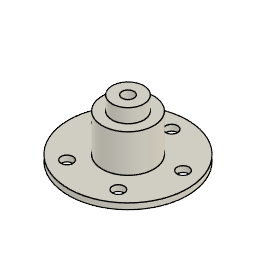
Brodie Stem Bolt (Autodesk Fusion 360 design; units mm, degrees)
Autodesk Fusion 360 part; units mm, degrees
sketch "Sketch1" plane through (0, 0, 0) normal (0, 0, 1) x (1, 0, 0)
  circle A0 centre (0, 0) radius 15
  constraint coincident A0.centre origin
extrude "Extrude1" add sketch "Sketch1" along normal blind 2
sketch "Sketch2" plane through (0, 0, 2) normal (0, 0, 1) x (-1, 0, 0)
  circle A0 centre (0, 0) radius 15
  circle A1 centre (0, -11) radius 1.5
  circle A2 centre (10.4616, -3.3992) radius 1.5
  circle A3 centre (6.4656, 8.8992) radius 1.5
  circle A4 centre (-6.4656, 8.8992) radius 1.5
  circle A5 centre (-10.4616, -3.3992) radius 1.5
  dimension "d4" = 360
extrude "Extrude2" cut sketch "Sketch2" against normal blind 19 contours A1 | A2 | A3 | A4 | A5
sketch "Sketch3" plane through (0, 0, 2) normal (0, 0, 1) x (-1, 0, 0)
  circle A0 centre (6.4656, 8.8992) radius 1.5
  circle A1 centre (10.4616, -3.3992) radius 1.5
  circle A2 centre (-6.4656, 8.8992) radius 1.5
  circle A3 centre (0, -11) radius 1.5
  circle A4 centre (-10.4616, -3.3992) radius 1.5
  circle A5 centre (0, 0) radius 15
  circle A6 centre (0, 0) radius 3
  constraint concentric A5 A6
extrude "Extrude3" cut sketch "Sketch3" against normal blind 2 contours A6
sketch "Sketch4" plane through (0, 0, 2) normal (0, 0, 1) x (-1, 0, 0)
  circle A0 centre (0, 0) radius 3
  circle A1 centre (6.4656, 8.8992) radius 1.5
  circle A2 centre (10.4616, -3.3992) radius 1.5
  circle A3 centre (-6.4656, 8.8992) radius 1.5
  circle A4 centre (0, -11) radius 1.5
  circle A5 centre (-10.4616, -3.3992) radius 1.5
  circle A6 centre (0, 0) radius 15
  circle A7 centre (0, 0) radius 6.5
  dimension "d9" = 13
  constraint concentric A0 A7
  measures "d9" diameter of A7
extrude "Extrude4" add sketch "Sketch4" along normal blind 9.5 contours A0 | A7
sketch "Sketch5" plane through (0, 0, 11.5) normal (0, 0, 1) x (-1, 0, 0)
  circle A0 centre (0, 0) radius 6.5
  circle A1 centre (0, 0) radius 4
  constraint coincident A0.centre A1.centre
extrude "Extrude5" add sketch "Sketch5" along normal blind 3.5 contours A1
sketch "Sketch6" plane through (0, 0, 2) normal (0, 0, -1) x (1, 0, 0)
  circle A0 centre (0, 0) radius 3
  circle A1 centre (0, 0) radius 1.5
  dimension "d14" = 3
  constraint coincident A0.centre A1.centre
  measures "d14" diameter of A1
extrude "Extrude6" cut sketch "Sketch6" against normal blind 100 contours A1
extrude "Extrude7" cut 1 faces at (-10.559, -3.3616, 0) along direction (0, 0, 1) blind 0.5
extrude "Extrude8" cut 1 faces at (-2.4832, 0.2236, 2) along direction (0, 0, 1) blind 0.5
